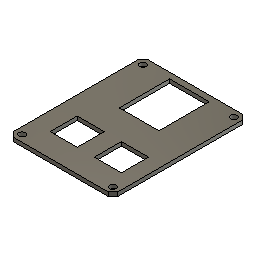
Secondary Board Plate v1 (Autodesk Fusion 360 design; units mm, degrees)
Autodesk Fusion 360 part; units mm, degrees
sketch "Sketch1" plane through (0, 0, 0) normal (0, 1, 0) x (1, 0, 0)
  line L0 (0, 0) -> (54, 0)
  line L1 (54, 0) -> (54, 69.5)
  line L2 (54, 69.5) -> (0, 69.5)
  line L3 (0, 69.5) -> (0, 0)
  dimension "d1" = 54
  dimension "d2" = 69.5
  constraint horizontal L0
  constraint vertical L1
  constraint horizontal L2
  constraint vertical L3
  constraint coincident L0.start L3.end
  measures "d1" distance of L0.start L0.end
  measures "d2" distance of L0.start L2.end
extrude "Extrude1" add sketch "Sketch1" along normal blind 2
chamfer "Chamfer1" distance 2.5 angle 45 4 edges at (54, 1, 0) (0, 1, 0) (54, 1, -69.5) (0, 1, -69.5)
sketch "Sketch2" plane through (0, 2, 0) normal (0, 1, 0) x (-1, 0, 0)
  line L0 (-2.5, -69.5) -> (0, -67)
  line L1 (0, -67) -> (0, -2.5)
  line L2 (0, -2.5) -> (-2.5, 0)
  line L3 (-2.5, 0) -> (-51.5, 0)
  line L4 (-51.5, 0) -> (-54, -2.5)
  line L5 (-54, -2.5) -> (-54, -67)
  line L6 (-54, -67) -> (-51.5, -69.5)
  line L7 (-51.5, -69.5) -> (-2.5, -69.5)
  line L8 (0, 0) -> (-3.5, 0)
  line L9 (-3.5, 0) -> (-3.5, -3.5)
  circle A0 centre (-3.5, -3.5) radius 1.625
  line L10 (-27, 0) -> (-27, -69.5)
  line L11 (0, -34.75) -> (-54, -34.75)
  circle A1 centre (-50.5, -3.5) radius 1.625
  circle A2 centre (-3.5, -66) radius 1.625
  circle A3 centre (-50.5, -66) radius 1.625
  dimension "d6" = 3.5
  dimension "d7" = 3.5
  dimension "d8" = 3.25
  constraint coincident L8.start origin
  constraint horizontal L8
  constraint perpendicular L8 L9
  constraint coincident L9.end A0.centre
  constraint midpoint L3 L10.start
  constraint midpoint L7 L10.end
  constraint midpoint L1 L11.start
  constraint midpoint L5 L11.end
  constraint symmetric A0 L10 A1
  constraint symmetric A0 L11 A2
  constraint symmetric L11 A1 A3
  measures "d6" distance of L8.start L8.end
  measures "d7" distance of L8.end L9.end
  measures "d8" diameter of A0
extrude "Extrude2" cut sketch "Sketch2" against normal blind 5 contours A0 | A1 | A2 | A3
sketch "Sketch3" plane through (0, 2, 0) normal (0, 1, 0) x (-1, 0, 0)
  circle A0 centre (-50.5, -3.5) radius 1.625
  circle A1 centre (-50.5, -66) radius 1.625
  circle A2 centre (-3.5, -3.5) radius 1.625
  circle A3 centre (-3.5, -66) radius 1.625
  line L0 (-2.5, -69.5) -> (0, -67)
  line L1 (0, -67) -> (0, -2.5)
  line L2 (0, -2.5) -> (-2.5, 0)
  line L3 (-2.5, 0) -> (-51.5, 0)
  line L4 (-51.5, 0) -> (-54, -2.5)
  line L5 (-54, -2.5) -> (-54, -67)
  line L6 (-54, -67) -> (-51.5, -69.5)
  line L7 (-51.5, -69.5) -> (-2.5, -69.5)
  line L8 (0, 0) -> (-16.5, 0)
  line L9 (-16.5, 0) -> (-16.5, -19)
  line L10 (-16.5, -19) -> (-39.35, -19)
  line L11 (-9.5, -12) -> (-23.5, -12)
  line L12 (-23.5, -12) -> (-23.5, -26)
  line L13 (-23.5, -26) -> (-9.5, -26)
  line L14 (-9.5, -26) -> (-9.5, -12)
  line L15 (-9.5, -12) -> (-23.5, -26) construction
  line L16 (-23.5, -12) -> (-9.5, -26) construction
  line L17 (-32.35, -26) -> (-46.35, -26)
  line L18 (-46.35, -26) -> (-46.35, -12)
  line L19 (-46.35, -12) -> (-32.35, -12)
  line L20 (-32.35, -12) -> (-32.35, -26)
  line L21 (-32.35, -26) -> (-46.35, -12) construction
  line L22 (-46.35, -26) -> (-32.35, -12) construction
  line L23 (0, 0) -> (-28.25, 0)
  line L24 (-28.25, 0) -> (-28.25, -40.5)
  line L25 (-28.25, -40.5) -> (-28.25, -66.5)
  line L26 (0, 0) -> (-18.25, 0)
  line L27 (-18.25, 0) -> (-18.25, -52)
  line L28 (-18.25, -52) -> (-16.75, -52)
  line L29 (-16.75, -52) -> (-28.25, -52)
  line L30 (-28.25, -52) -> (-28.25, -66.5)
  line L31 (-28.25, -66.5) -> (-16.75, -66.5)
  line L32 (-16.75, -66.5) -> (-16.75, -52)
  line L33 (-16.75, -52) -> (-28.25, -52)
  line L34 (-28.25, -52) -> (-28.25, -40.5)
  line L35 (-28.25, -40.5) -> (-16.75, -40.5)
  line L36 (-16.75, -40.5) -> (-16.75, -52)
  line L37 (0, 0) -> (-35.75, 0)
  line L38 (-35.75, 0) -> (-35.75, -44.5)
  line L39 (-35.75, -44.5) -> (-37.25, -44.5)
  line L40 (-37.25, -44.5) -> (-28.25, -44.5)
  line L41 (-28.25, -44.5) -> (-28.25, -40.5)
  line L42 (-28.25, -40.5) -> (-37.25, -40.5)
  line L43 (-37.25, -40.5) -> (-37.25, -44.5)
  line L44 (-37.25, -44.5) -> (-28.25, -44.5)
  line L45 (-28.25, -44.5) -> (-28.25, -66.5)
  line L46 (-28.25, -66.5) -> (-37.25, -66.5)
  line L47 (-37.25, -66.5) -> (-37.25, -44.5)
  point P0 (-16.5, -19)
  point P1 (-39.35, -19)
  dimension "d11" = 16.5
  dimension "d12" = 19
  dimension "d13" = 22.85
  dimension "d14" = 14
  dimension "d15" = 14
  dimension "d16" = 14
  dimension "d17" = 14
  dimension "d18" = 28.25
  dimension "d19" = 40.5
  dimension "d20" = 26
  dimension "d21" = 18.25
  dimension "d22" = 52
  dimension "d23" = 1.5
  dimension "d24" = 35.75
  dimension "d25" = 44.5
  dimension "d26" = 1.5
  constraint coincident L8.start L23.start
  constraint perpendicular L1 L8
  constraint perpendicular L8 L9
  constraint perpendicular L9 L10
  constraint horizontal L11
  constraint perpendicular L11 L12
  constraint parallel L11 L13
  constraint parallel L12 L14
  constraint coincident L15 P0
  constraint coincident L16 P0
  constraint coincident P0 L9.end
  constraint horizontal L17
  constraint perpendicular L17 L18
  constraint parallel L17 L19
  constraint parallel L18 L20
  constraint coincident L21 P1
  constraint coincident L22 P1
  constraint coincident P1 L10.end
  constraint perpendicular L9 L23
  constraint perpendicular L10 L24
  constraint parallel L24 L25
  constraint parallel L23 L26
  constraint perpendicular L13 L27
  constraint perpendicular L27 L28
  constraint horizontal L29
  constraint vertical L30
  constraint horizontal L31
  constraint vertical L32
  constraint horizontal L33
  constraint vertical L34
  constraint horizontal L35
  constraint vertical L36
  constraint perpendicular L24 L37
  constraint perpendicular L17 L38
  constraint perpendicular L38 L39
  constraint horizontal L40
  constraint vertical L41
  constraint horizontal L42
  constraint vertical L43
  constraint horizontal L44
  constraint vertical L45
  constraint horizontal L46
  constraint vertical L47
  measures "d11" distance of L8.start L8.end
  measures "d12" distance of L8.end P0
  measures "d13" distance of P0 P1
  measures "d14" distance of L12.end L13.end
  measures "d15" distance of L11.end L12.end
  measures "d16" distance of L18.end L19.end
  measures "d17" distance of L17.end L18.end
  measures "d18" distance of L8.start L23.end
  measures "d19" distance of L23.end L24.end
  measures "d20" distance of L24.end L25.end
  measures "d21" distance of L8.start L26.end
  measures "d22" distance of L26.end L27.end
  measures "d23" distance of L27.end L28.end
  measures "d24" distance of L8.start L37.end
  measures "d25" distance of L37.end L38.end
  measures "d26" distance of L38.end L39.end
extrude "Extrude3" cut sketch "Sketch3" against normal blind 2 contours L9 L10 L11 L13 L14 L27 | L9 L10 L11 L27 | L10 L11 L12 L27 | L17 L18 L19 L38 | L10 L19 L20 L38 | L10 L12 L13 L27 | L10 L17 L20 L38 | L25 L27 L29 L33 L34 L35 L41 L45 | L25 L34 L38 L40 L41 L42 L44 | L25 L30 L34 L39 L40 L44 L45 L46 L47 | L27 L28 L29 L33 L35 L36 | L38 L39 L40 L42 L43 L44 | L25 L28 L29 L30 L31 L32 L33 L45
equation "d13 = 39.35 mm - 16.5 mm"
equation "d19 = 42 mm - 1.5 mm"
